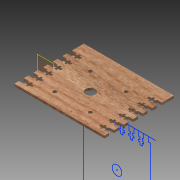
# Autodesk Inventor part: stepperMotorMountPlate01
Saved by Autodesk Inventor 2013 (Build 170138000, 138)
## iProperties
Created: 2013-02-23
Part Number: stepperMotorMountPlate01
Material: Wood (Birch)
Document SubType Name: Modeling
Designer: Nano
Density: 0.55 g/cm^3
Mass: 20.9125 g
Surface Area: 257.148 cm^2
Volume: 38.0226 cm^3
Author: Nano
Autodesk Inventor part; units mm, degrees
ref_plane "YZ Plane" through (0, 0, 0) normal (1, 0, 0) x (0, 1, 0)
ref_plane "XZ Plane" through (0, 0, 0) normal (0, 1, 0) x (-1, 0, 0)
ref_plane "XY Plane" through (0, 0, 0) normal (0, 0, 1) x (1, 0, 0)
sketch "Sketch1" plane through (0, 0, 0) normal (0, 1, 0) x (-1, 0, 0)
  circle A0 centre (0, 0) radius 3.556
  line L0 (59.5312, 50.8) -> (-59.5312, 50.8)
  line L1 (-59.5312, 50.8) -> (-59.5312, -50.8)
  line L2 (-59.5312, -50.8) -> (59.5312, -50.8)
  line L3 (59.5312, -50.8) -> (59.5312, 50.8)
  line L4 (59.5312, 50.8) -> (-59.5312, -50.8) construction
  line L5 (-59.5312, 50.8) -> (59.5312, -50.8) construction
  line L6 (0, 0) -> (71.842, -71.842)
  line L7 (0, 0) -> (101.6, 0) construction
  circle A1 centre (23.5732, -23.5732) radius 2.3813
  circle A2 centre (23.5732, 23.5732) radius 2.3813
  circle A3 centre (-23.5732, 23.5732) radius 2.3813
  circle A4 centre (-23.5732, -23.5732) radius 2.3813
  dimension "d0" = 7.112
  dimension "d1" = 119.0625
  dimension "d2" = 101.6
  dimension "d3" = 101.6
  dimension "d4" = 45
  dimension "d5" = 4.7625
  dimension "d6" = 33.3375
  dimension "d9" = 360
  constraints: 16 end point, 5 centre point, 2 midpoint, 2 parallel, 1 equal length, 1 horizontal, 1 perpendicular, 9 other
  measures "d0" diameter of A0
  measures "d1" distance of L0.start L0.end
  measures "d2" distance of L1.end L0.end
  measures "d3" distance of L6.start L6.end
  measures "d4" angle of L6 L7
  measures "d5" diameter of A1
  measures "d6" distance of L6.start A1.centre
extrude "Extrusion1" add sketch "Sketch1" along normal blind 3.175
ref_plane "Work Plane1" through (-59.5312, 0, 0) normal (0, 0, 1) x (1, 0, 0)
sketch "Sketch4" plane through (0, 0, 0) normal (0, -1, 0) x (1, 0, 0)
  line L0 (-59.5312, 50.8) -> (59.5312, 50.8)
  line L1 (59.5312, 50.8) -> (59.5312, 41.0053)
  line L2 (59.5312, 41.0053) -> (-59.5312, 41.0053)
  line L3 (-59.5312, 41.0053) -> (-59.5312, 50.8)
  constraints: 8 end point, 2 parallel, 1 horizontal, 1 perpendicular
extrude "Extrusion4" cut sketch "Sketch4" against normal through all
sketch "Sketch5" plane through (0, 3.175, 0) normal (0, 1, 0) x (1, 0, 0)
  line L0 (59.5312, -41.0053) -> (59.5312, 50.8) projected
  line L1 (-59.5312, 50.8) -> (-59.5312, -41.0053) projected
  circle A0 centre (0, 0) radius 3.556 projected
  line L2 (53.1813, -33.3375) -> (50.4031, -33.3375) projected
  line L3 (50.4031, -33.3375) -> (50.4031, -35.7187) projected
  line L4 (50.4031, -35.7187) -> (47.2281, -35.7187) projected
  line L5 (47.2281, -35.7187) -> (47.2281, -33.3375) projected
  line L6 (47.2281, -33.3375) -> (44.2913, -33.3375) projected
  line L7 (44.2913, -33.3375) -> (44.2913, -30.1625) projected
  line L8 (44.2913, -30.1625) -> (47.2281, -30.1625) projected
  line L9 (47.2281, -30.1625) -> (47.2281, -27.7812) projected
  line L10 (47.2281, -27.7812) -> (50.4031, -27.7812) projected
  line L11 (50.4031, -27.7812) -> (50.4031, -30.1625) projected
  line L12 (50.4031, -30.1625) -> (53.1813, -30.1625) projected
  line L13 (53.1813, -30.1625) -> (53.1813, -28.575) projected
  line L14 (53.1813, -28.575) -> (59.5313, -28.575) projected
  line L15 (59.5313, -22.225) -> (59.5313, -28.575) projected
  line L16 (59.5313, -22.225) -> (53.1813, -22.225) projected
  line L17 (53.1813, -22.225) -> (53.1813, -20.6375) projected
  line L18 (53.1813, -20.6375) -> (50.4031, -20.6375) projected
  line L19 (50.4031, -20.6375) -> (50.4031, -23.0187) projected
  line L20 (50.4031, -23.0187) -> (47.2281, -23.0187) projected
  line L21 (47.2281, -23.0187) -> (47.2281, -20.6375) projected
  line L22 (47.2281, -20.6375) -> (44.2913, -20.6375) projected
  line L23 (44.2913, -20.6375) -> (44.2913, -17.4625) projected
  line L24 (44.2913, -17.4625) -> (47.2281, -17.4625) projected
  line L25 (47.2281, -17.4625) -> (47.2281, -15.0812) projected
  line L26 (47.2281, -15.0812) -> (50.4031, -15.0812) projected
  line L27 (50.4031, -15.0812) -> (50.4031, -17.4625) projected
  line L28 (50.4031, -17.4625) -> (53.1813, -17.4625) projected
  line L29 (53.1813, -17.4625) -> (53.1813, -15.875) projected
  line L30 (53.1813, -15.875) -> (59.5313, -15.875) projected
  line L31 (59.5313, -9.525) -> (59.5313, -15.875) projected
  line L32 (59.5313, -9.525) -> (53.1813, -9.525) projected
  line L33 (53.1813, -9.525) -> (53.1813, -7.9375) projected
  line L34 (53.1813, -7.9375) -> (50.4031, -7.9375) projected
  line L35 (50.4031, -7.9375) -> (50.4031, -10.3187) projected
  line L36 (50.4031, -10.3187) -> (47.2281, -10.3187) projected
  line L37 (47.2281, -10.3187) -> (47.2281, -7.9375) projected
  line L38 (47.2281, -7.9375) -> (44.2913, -7.9375) projected
  line L39 (44.2913, -7.9375) -> (44.2913, -4.7625) projected
  line L40 (44.2913, -4.7625) -> (47.2281, -4.7625) projected
  line L41 (47.2281, -4.7625) -> (47.2281, -2.3812) projected
  line L42 (47.2281, -2.3812) -> (50.4031, -2.3812) projected
  line L43 (50.4031, -2.3812) -> (50.4031, -4.7625) projected
  line L44 (50.4031, -4.7625) -> (53.1813, -4.7625) projected
  line L45 (53.1813, -4.7625) -> (53.1813, -3.175) projected
  line L46 (53.1813, -3.175) -> (59.5313, -3.175) projected
  line L47 (59.5313, 3.175) -> (59.5313, -3.175) projected
  line L48 (59.5313, 3.175) -> (53.1813, 3.175) projected
  line L49 (53.1813, 3.175) -> (53.1813, 4.7625) projected
  line L50 (53.1813, 4.7625) -> (50.4031, 4.7625) projected
  line L51 (50.4031, 4.7625) -> (50.4031, 2.3813) projected
  line L52 (50.4031, 2.3813) -> (47.2281, 2.3813) projected
  line L53 (47.2281, 2.3813) -> (47.2281, 4.7625) projected
  line L54 (47.2281, 4.7625) -> (44.2913, 4.7625) projected
  line L55 (44.2913, 4.7625) -> (44.2913, 7.9375) projected
  line L56 (44.2913, 7.9375) -> (47.2281, 7.9375) projected
  line L57 (47.2281, 7.9375) -> (47.2281, 10.3188) projected
  line L58 (47.2281, 10.3188) -> (50.4031, 10.3188) projected
  line L59 (50.4031, 10.3188) -> (50.4031, 7.9375) projected
  line L60 (50.4031, 7.9375) -> (53.1813, 7.9375) projected
  line L61 (53.1813, 7.9375) -> (53.1813, 9.525) projected
  line L62 (53.1813, 9.525) -> (59.5313, 9.525) projected
  line L63 (59.5313, 15.875) -> (59.5313, 9.525) projected
  line L64 (59.5313, 15.875) -> (53.1813, 15.875) projected
  line L65 (53.1813, 15.875) -> (53.1813, 17.4625) projected
  line L66 (53.1813, 17.4625) -> (50.4031, 17.4625) projected
  line L67 (50.4031, 17.4625) -> (50.4031, 15.0813) projected
  line L68 (50.4031, 15.0813) -> (47.2281, 15.0813) projected
  line L69 (47.2281, 15.0813) -> (47.2281, 17.4625) projected
  line L70 (47.2281, 17.4625) -> (44.2913, 17.4625) projected
  line L71 (44.2913, 17.4625) -> (44.2913, 20.6375) projected
  line L72 (44.2913, 20.6375) -> (47.2281, 20.6375) projected
  line L73 (47.2281, 20.6375) -> (47.2281, 23.0188) projected
  line L74 (47.2281, 23.0188) -> (50.4031, 23.0188) projected
  line L75 (50.4031, 23.0188) -> (50.4031, 20.6375) projected
  line L76 (50.4031, 20.6375) -> (53.1813, 20.6375) projected
  line L77 (53.1813, 20.6375) -> (53.1813, 22.225) projected
  line L78 (53.1813, 22.225) -> (59.5313, 22.225) projected
  line L79 (59.5313, 28.575) -> (59.5313, 22.225) projected
  line L80 (59.5313, 28.575) -> (53.1813, 28.575) projected
  line L81 (53.1813, 28.575) -> (53.1813, 30.1625) projected
  line L82 (53.1813, 30.1625) -> (50.4031, 30.1625) projected
  line L83 (50.4031, 30.1625) -> (50.4031, 27.7813) projected
  line L84 (50.4031, 27.7813) -> (47.2281, 27.7813) projected
  line L85 (47.2281, 27.7813) -> (47.2281, 30.1625) projected
  line L86 (47.2281, 30.1625) -> (44.2913, 30.1625) projected
  line L87 (44.2913, 30.1625) -> (44.2913, 33.3375) projected
  line L88 (44.2913, 33.3375) -> (47.2281, 33.3375) projected
  line L89 (47.2281, 33.3375) -> (47.2281, 35.7188) projected
  line L90 (47.2281, 35.7188) -> (50.4031, 35.7188) projected
  line L91 (50.4031, 35.7188) -> (50.4031, 33.3375) projected
  line L92 (50.4031, 33.3375) -> (53.1813, 33.3375) projected
  line L93 (53.1813, 33.3375) -> (53.1813, 34.925) projected
  line L94 (53.1813, 34.925) -> (59.5313, 34.925) projected
  line L95 (59.5313, 41.275) -> (59.5313, 34.925) projected
  line L96 (59.5313, 41.275) -> (53.1813, 41.275) projected
  line L97 (53.1813, 41.275) -> (53.1813, 44.45) projected
  line L98 (-53.1813, 44.45) -> (53.1813, 44.45) projected
  line L99 (-53.1813, 44.45) -> (-53.1813, 41.275) projected
  line L100 (-53.1813, 41.275) -> (-59.5312, 41.275) projected
  line L101 (-59.5312, 34.925) -> (-59.5312, 41.275) projected
  line L102 (-59.5312, 34.925) -> (-53.1813, 34.925) projected
  line L103 (-53.1813, 34.925) -> (-53.1813, 33.3375) projected
  line L104 (-53.1813, 33.3375) -> (-50.4031, 33.3375) projected
  line L105 (-50.4031, 33.3375) -> (-50.4031, 35.7188) projected
  line L106 (-50.4031, 35.7188) -> (-47.2281, 35.7188) projected
  line L107 (-47.2281, 35.7188) -> (-47.2281, 33.3375) projected
  line L108 (-47.2281, 33.3375) -> (-44.2912, 33.3375) projected
  line L109 (-44.2912, 33.3375) -> (-44.2912, 30.1625) projected
  line L110 (-44.2912, 30.1625) -> (-47.2281, 30.1625) projected
  line L111 (-47.2281, 30.1625) -> (-47.2281, 27.7813) projected
  line L112 (-47.2281, 27.7813) -> (-50.4031, 27.7813) projected
  line L113 (-50.4031, 27.7813) -> (-50.4031, 30.1625) projected
  line L114 (-50.4031, 30.1625) -> (-53.1813, 30.1625) projected
  line L115 (-53.1813, 30.1625) -> (-53.1813, 28.575) projected
  line L116 (-53.1813, 28.575) -> (-59.5312, 28.575) projected
  line L117 (-59.5312, 22.225) -> (-59.5312, 28.575) projected
  line L118 (-59.5312, 22.225) -> (-53.1813, 22.225) projected
  line L119 (-53.1813, 22.225) -> (-53.1813, 20.6375) projected
  line L120 (-53.1813, 20.6375) -> (-50.4031, 20.6375) projected
  line L121 (-50.4031, 20.6375) -> (-50.4031, 23.0188) projected
  line L122 (-50.4031, 23.0188) -> (-47.2281, 23.0188) projected
  line L123 (-47.2281, 23.0188) -> (-47.2281, 20.6375) projected
  line L124 (-47.2281, 20.6375) -> (-44.2912, 20.6375) projected
  line L125 (-44.2912, 20.6375) -> (-44.2912, 17.4625) projected
  line L126 (-44.2912, 17.4625) -> (-47.2281, 17.4625) projected
  line L127 (-47.2281, 17.4625) -> (-47.2281, 15.0813) projected
  line L128 (-47.2281, 15.0813) -> (-50.4031, 15.0813) projected
  line L129 (-50.4031, 15.0813) -> (-50.4031, 17.4625) projected
  line L130 (-50.4031, 17.4625) -> (-53.1813, 17.4625) projected
  line L131 (-53.1813, 17.4625) -> (-53.1813, 15.875) projected
  line L132 (-53.1813, 15.875) -> (-59.5312, 15.875) projected
  line L133 (-59.5312, 9.525) -> (-59.5312, 15.875) projected
  line L134 (-59.5312, 9.525) -> (-53.1813, 9.525) projected
  line L135 (-53.1813, 9.525) -> (-53.1813, 7.9375) projected
  line L136 (-53.1813, 7.9375) -> (-50.4031, 7.9375) projected
  line L137 (-50.4031, 7.9375) -> (-50.4031, 10.3188) projected
  line L138 (-50.4031, 10.3188) -> (-47.2281, 10.3188) projected
  line L139 (-47.2281, 10.3188) -> (-47.2281, 7.9375) projected
  line L140 (-47.2281, 7.9375) -> (-44.2912, 7.9375) projected
  line L141 (-44.2912, 7.9375) -> (-44.2912, 4.7625) projected
  line L142 (-44.2912, 4.7625) -> (-47.2281, 4.7625) projected
  line L143 (-47.2281, 4.7625) -> (-47.2281, 2.3813) projected
  line L144 (-47.2281, 2.3813) -> (-50.4031, 2.3813) projected
  line L145 (-50.4031, 2.3813) -> (-50.4031, 4.7625) projected
  line L146 (-50.4031, 4.7625) -> (-53.1813, 4.7625) projected
  line L147 (-53.1813, 4.7625) -> (-53.1813, 3.175) projected
  line L148 (-53.1813, 3.175) -> (-59.5312, 3.175) projected
  line L149 (-59.5312, -3.175) -> (-59.5312, 3.175) projected
  line L150 (-59.5312, -3.175) -> (-53.1813, -3.175) projected
  line L151 (-53.1813, -3.175) -> (-53.1813, -4.7625) projected
  line L152 (-53.1813, -4.7625) -> (-50.4031, -4.7625) projected
  line L153 (-50.4031, -4.7625) -> (-50.4031, -2.3812) projected
  line L154 (-50.4031, -2.3812) -> (-47.2281, -2.3812) projected
  line L155 (-47.2281, -2.3812) -> (-47.2281, -4.7625) projected
  line L156 (-47.2281, -4.7625) -> (-44.2912, -4.7625) projected
  line L157 (-44.2912, -4.7625) -> (-44.2912, -7.9375) projected
  line L158 (-44.2912, -7.9375) -> (-47.2281, -7.9375) projected
  line L159 (-47.2281, -7.9375) -> (-47.2281, -10.3187) projected
  line L160 (-47.2281, -10.3187) -> (-50.4031, -10.3187) projected
  line L161 (-50.4031, -10.3187) -> (-50.4031, -7.9375) projected
  line L162 (-50.4031, -7.9375) -> (-53.1813, -7.9375) projected
  line L163 (-53.1813, -7.9375) -> (-53.1813, -9.525) projected
  line L164 (-53.1813, -9.525) -> (-59.5312, -9.525) projected
  line L165 (-59.5312, -15.875) -> (-59.5312, -9.525) projected
  line L166 (-59.5312, -15.875) -> (-53.1813, -15.875) projected
  line L167 (-53.1813, -15.875) -> (-53.1813, -17.4625) projected
  line L168 (-53.1813, -17.4625) -> (-50.4031, -17.4625) projected
  line L169 (-50.4031, -17.4625) -> (-50.4031, -15.0812) projected
  line L170 (-50.4031, -15.0812) -> (-47.2281, -15.0812) projected
  line L171 (-47.2281, -15.0812) -> (-47.2281, -17.4625) projected
  line L172 (-47.2281, -17.4625) -> (-44.2912, -17.4625) projected
  line L173 (-44.2912, -17.4625) -> (-44.2912, -20.6375) projected
  line L174 (-44.2912, -20.6375) -> (-47.2281, -20.6375) projected
  line L175 (-47.2281, -20.6375) -> (-47.2281, -23.0187) projected
  line L176 (-47.2281, -23.0187) -> (-50.4031, -23.0187) projected
  line L177 (-50.4031, -23.0187) -> (-50.4031, -20.6375) projected
  line L178 (-50.4031, -20.6375) -> (-53.1813, -20.6375) projected
  line L179 (-53.1813, -20.6375) -> (-53.1813, -22.225) projected
  line L180 (-53.1813, -22.225) -> (-59.5312, -22.225) projected
  line L181 (-59.5312, -28.575) -> (-59.5312, -22.225) projected
  line L182 (-59.5312, -28.575) -> (-53.1813, -28.575) projected
  line L183 (-53.1813, -28.575) -> (-53.1813, -30.1625) projected
  line L184 (-53.1813, -30.1625) -> (-50.4031, -30.1625) projected
  line L185 (-50.4031, -30.1625) -> (-50.4031, -27.7812) projected
  line L186 (-50.4031, -27.7812) -> (-47.2281, -27.7812) projected
  line L187 (-47.2281, -27.7812) -> (-47.2281, -30.1625) projected
  line L188 (-47.2281, -30.1625) -> (-44.2912, -30.1625) projected
  line L189 (-44.2912, -30.1625) -> (-44.2912, -33.3375) projected
  line L190 (-44.2912, -33.3375) -> (-47.2281, -33.3375) projected
  line L191 (-47.2281, -33.3375) -> (-47.2281, -35.7187) projected
  line L192 (-47.2281, -35.7187) -> (-50.4031, -35.7187) projected
  line L193 (-50.4031, -35.7187) -> (-50.4031, -33.3375) projected
  line L194 (-50.4031, -33.3375) -> (-53.1813, -33.3375) projected
  line L195 (-53.1813, -33.3375) -> (-53.1813, -34.925) projected
  line L196 (-53.1813, -34.925) -> (-59.5312, -34.925) projected
  line L197 (-59.5312, -41.275) -> (-59.5312, -34.925) projected
  line L198 (-59.5312, -41.275) -> (-53.1813, -41.275) projected
  line L199 (-53.1813, -41.275) -> (-53.1813, -44.45) projected
  line L200 (53.1813, -44.45) -> (-53.1813, -44.45) projected
  line L201 (53.1813, -44.45) -> (53.1813, -41.275) projected
  line L202 (53.1813, -41.275) -> (59.5313, -41.275) projected
  line L203 (59.5313, -34.925) -> (59.5313, -41.275) projected
  line L204 (59.5313, -34.925) -> (53.1813, -34.925) projected
  line L205 (53.1813, -34.925) -> (53.1813, -33.3375) projected
  circle A1 centre (0, 0) radius 5.9531 projected
  constraints: 2 other
extrude "Extrusion5" cut sketch "Sketch5" against normal blind 25.4 contours L204 L205 L2 L3 L4 L5 L6 L7 L8 L9 L10 L11 L12 L13 L14 L0 | L16 L17 L18 L19 L20 L21 L22 L23 L24 L25 L26 L27 L28 L29 L30 L0 | L32 L33 L34 L35 L36 L37 L38 L39 L40 L41 L42 L43 L44 L45 L46 L0 | L48 L49 L50 L51 L52 L53 L54 L55 L56 L57 L58 L59 L60 L61 L62 L0 | L1 L182 L183 L184 L185 L186 L187 L188 L189 L190 L191 L192 L193 L194 L195 L196 | L64 L65 L66 L67 L68 L69 L70 L71 L72 L73 L74 L75 L76 L77 L78 L0 | L1 L166 L167 L168 L169 L170 L171 L172 L173 L174 L175 L176 L177 L178 L179 L180 | L80 L81 L82 L83 L84 L85 L86 L87 L88 L89 L90 L91 L92 L93 L94 L0 | L1 L150 L151 L152 L153 L154 L155 L156 L157 L158 L159 L160 L161 L162 L163 L164 | L1 L134 L135 L136 L137 L138 L139 L140 L141 L142 L143 L144 L145 L146 L147 L148 | L1 L118 L119 L120 L121 L122 L123 L124 L125 L126 L127 L128 L129 L130 L131 L132 | L1 L102 L103 L104 L105 L106 L107 L108 L109 L110 L111 L112 L113 L114 L115 L116 | A1
body "Solid1"
